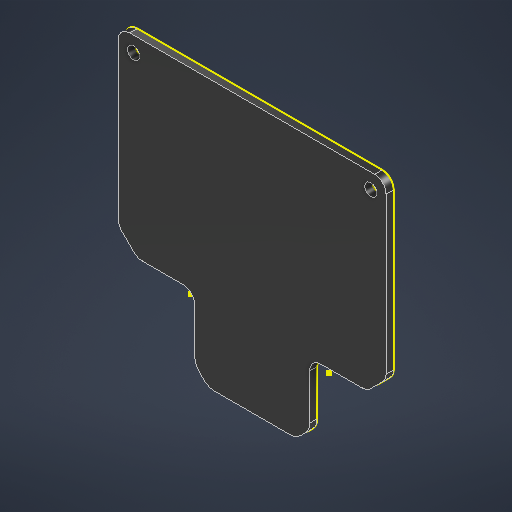
# Autodesk Inventor part: Motor Driver Board
Saved by Autodesk Inventor 2026.1 (Build 301233020, 233B)
## iProperties
Created: 2026-04-03
Part Number: Motor Driver Board
Material: Generic
Document SubType Name: Modeling
Designer: Bahaa
Density: 1 g/cm^3
Appearance: Glossy - Black
Mass: 8.08903 g
Surface Area: 86.5661 cm^2
Volume: 8.08903 cm^3
Author: Bahaa
Autodesk Inventor part; units mm, degrees
ref_plane "YZ Plane" through (0, 0, 0) normal (1, 0, 0) x (0, 1, 0)
ref_plane "XZ Plane" through (0, 0, 0) normal (0, 1, 0) x (-1, 0, 0)
ref_plane "XY Plane" through (0, 0, 0) normal (0, 0, 1) x (1, 0, 0)
sketch "Sketch1" plane through (0, 0, 0) normal (0, 1, 0) x (-1, 0, 0)
  line L0 (35, 25) -> (-35, 25)
  line L1 (-35, 25) -> (-35, -20)
  line L2 (-30, -25) -> (30, -25)
  line L3 (35, -20) -> (35, 25)
  line L4 (35, 25) -> (-35, -25) construction
  line L5 (-35, 25) -> (35, -25) construction
  line L6 (35, 25) -> (31, 25)
  line L7 (31, 25) -> (31, 21) construction
  line L8 (31, 21) -> (35, 21) construction
  line L9 (35, 21) -> (35, 25)
  line L10 (0, 25) -> (0, -25) construction
  circle A0 centre (31, 21) radius 1.6
  circle A1 centre (-31, 21) radius 1.6
  line L11 (15, -45) -> (-15, -45)
  line L12 (-15, -45) -> (-15, -5)
  line L13 (-15, -5) -> (15, -5)
  line L14 (15, -5) -> (15, -45)
  line L15 (15, -45) -> (-15, -5) construction
  line L16 (-15, -45) -> (15, -5) construction
  line L17 (27, 17) -> (35, 17) construction
  line L18 (35, 17) -> (35, 25) construction
  line L19 (35, 25) -> (27, 25) construction
  line L20 (27, 25) -> (27, 17) construction
  line L21 (27, 17) -> (35, 25) construction
  line L22 (35, 17) -> (27, 25) construction
  line L23 (-27, 17) -> (-35, 17) construction
  line L24 (-35, 17) -> (-35, 25) construction
  line L25 (-35, 25) -> (-27, 25) construction
  line L26 (-27, 25) -> (-27, 17) construction
  line L27 (-27, 17) -> (-35, 25) construction
  line L28 (-35, 17) -> (-27, 25) construction
  line L29 (35, -20) -> (30, -25)
  line L30 (-30, -25) -> (-35, -20)
  point P0 (0, 0)
  point P1 (15, -25)
  point P2 (-15, -25)
  dimension "d0" = 70
  dimension "d1" = 50
  dimension "d11" = 4
  dimension "d12" = 4
  dimension "d13" = 3.2
  dimension "d14" = 30
  dimension "d15" = 40
  dimension "d16" = 5
  dimension "d17" = 5
  dimension "d18" = 5
  dimension "d19" = 5
  constraints: 62 end point, 10 midpoint, 10 parallel, 5 horizontal, 5 perpendicular, 4 point on line, 2 centre point, 2 coincident, 1 symmetric about line, 1 other
  measures "d0" distance of L5.end L4.end
  measures "d1" distance of L4.end L0.end
  measures "d11" distance of L8.end L7.end
  measures "d12" distance of L7.end L6.end
  measures "d13" diameter of A0
  measures "d14" distance between parallel lines of L12 L14
  measures "d15" distance of L11.end L12.end
  measures "d16" distance of L3.start L5.end
  measures "d17" distance of L2.end L5.end
  measures "d18" distance of L2.start L4.end
  measures "d19" distance of L1.end L4.end
extrude "Extrusion1" add sketch "Sketch1" along normal blind 2
fillet "Fillet1" radius 3 8 edges at (-35, 1, 25) (35, 1, 25) (-15, 1, -25) (15, 1, -25) (30, 1, -25) (35, 1, -20) (-35, 1, -20) (-30, 1, -25)
chamfer "Chamfer1" distance 3.5 angle 45 2 edges at (-15, 1, -45) (15, 1, -45)
fillet "Fillet3" radius 4 4 edges at (15, 1, -41.5) (11.5, 1, -45) (-11.5, 1, -45) (-15, 1, -41.5)
sketch "Sketch2" plane through (0, 2, 0) normal (0, 1, 0) x (1, 0, 0)
  arc A0 (-9.8431, 45) -> (-12.6716, 43.8284) centre (-9.8431, 41) ccw projected
  line L0 (-9.8431, 45) -> (9.8431, 45) projected
  arc A1 (12.6716, 43.8284) -> (9.8431, 45) centre (9.8431, 41) ccw projected
  line L1 (12.6716, 43.8284) -> (13.8284, 42.6716) projected
  arc A2 (15, 39.8431) -> (13.8284, 42.6716) centre (11, 39.8431) ccw projected
  line L2 (15, 39.8431) -> (15, 28) projected
  arc A3 (15, 28) -> (18, 25) centre (18, 28) ccw projected
  line L3 (18, 25) -> (28.7574, 25) projected
  arc A4 (30.8787, 24.1213) -> (28.7574, 25) centre (28.7574, 22) ccw projected
  line L4 (30.8787, 24.1213) -> (34.1213, 20.8787) projected
  arc A5 (35, 18.7574) -> (34.1213, 20.8787) centre (32, 18.7574) ccw projected
  line L5 (35, 18.7574) -> (35, -22) projected
  arc A6 (32, -25) -> (35, -22) centre (32, -22) ccw projected
  line L6 (32, -25) -> (-32, -25) projected
  arc A7 (-35, -22) -> (-32, -25) centre (-32, -22) ccw projected
  line L7 (-35, -22) -> (-35, 18.7574) projected
  arc A8 (-34.1213, 20.8787) -> (-35, 18.7574) centre (-32, 18.7574) ccw projected
  line L8 (-34.1213, 20.8787) -> (-30.8787, 24.1213) projected
  arc A9 (-28.7574, 25) -> (-30.8787, 24.1213) centre (-28.7574, 22) ccw projected
  line L9 (-28.7574, 25) -> (-18, 25) projected
  arc A10 (-18, 25) -> (-15, 28) centre (-18, 28) ccw projected
  line L10 (-15, 28) -> (-15, 39.8431) projected
  arc A11 (-13.8284, 42.6716) -> (-15, 39.8431) centre (-11, 39.8431) ccw projected
  line L11 (-13.8284, 42.6716) -> (-12.6716, 43.8284) projected
  circle A12 centre (31, -21) radius 1.6 projected
  circle A13 centre (-31, -21) radius 1.6 projected
  point P0 (0, 0)
equation "\"d17\" = d16"
equation "\"d18\" = d16"
equation "\"d19\" = d18"
body "Solid1"
